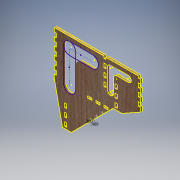
# Autodesk Inventor part: ArmSide
Saved by Autodesk Inventor 2019 (Build 230136000, 136)
## iProperties
Created: 2019-01-17
Part Number: ArmSide
Material: Wood (Birch)
Document SubType Name: Modeling
Designer: nxgam
Density: 0.55 g/cm^3
Appearance: Birch - Natural Polished
Mass: 65.7637 g
Surface Area: 562.081 cm^2
Volume: 119.57 cm^3
Author: nxgam
Autodesk Inventor part; units mm, degrees
(part 1 of 2)
ref_plane "YZ Plane" through (0, 0, 0) normal (1, 0, 0) x (0, 1, 0)
ref_plane "XZ Plane" through (0, 0, 0) normal (0, 1, 0) x (-1, 0, 0)
ref_plane "XY Plane" through (0, 0, 0) normal (0, 0, 1) x (1, 0, 0)
sketch "Sketch1" plane through (0, 0, 0) normal (0, 0, 1) x (1, 0, 0)
  line L0 (0, 0) -> (76.2, 0)
  line L1 (76.2, 0) -> (76.2, 579.12)
  line L2 (76.2, 579.12) -> (0, 579.12)
  line L3 (0, 579.12) -> (0, 0)
  line L4 (0, 568.96) -> (5.08, 568.96)
  line L5 (5.08, 568.96) -> (5.08, 558.8)
  line L6 (5.08, 558.8) -> (0, 558.8)
  line L7 (0, 558.8) -> (0, 568.96)
  line L8 (0, 548.64) -> (5.08, 548.64)
  line L9 (5.08, 548.64) -> (5.08, 538.48)
  line L10 (5.08, 538.48) -> (0, 538.48)
  line L11 (0, 538.48) -> (0, 548.64)
  line L12 (0, 558.8) -> (0, -20.32)
  line L13 (0, 528.32) -> (5.08, 528.32)
  line L14 (5.08, 528.32) -> (5.08, 518.16)
  line L15 (5.08, 518.16) -> (0, 518.16)
  line L16 (0, 518.16) -> (0, 528.32)
  line L17 (0, 538.48) -> (0, -40.64)
  line L18 (0, 508) -> (5.08, 508)
  line L19 (5.08, 508) -> (5.08, 497.84)
  line L20 (5.08, 497.84) -> (0, 497.84)
  line L21 (0, 497.84) -> (0, 508)
  line L22 (0, 518.16) -> (0, -60.96)
  line L23 (0, 487.68) -> (5.08, 487.68)
  line L24 (5.08, 487.68) -> (5.08, 477.52)
  line L25 (5.08, 477.52) -> (0, 477.52)
  line L26 (0, 477.52) -> (0, 487.68)
  line L27 (0, 497.84) -> (0, -81.28)
  line L28 (0, 467.36) -> (5.08, 467.36)
  line L29 (5.08, 467.36) -> (5.08, 457.2)
  line L30 (5.08, 457.2) -> (0, 457.2)
  line L31 (0, 457.2) -> (0, 467.36)
  line L32 (0, 477.52) -> (0, -101.6)
  line L33 (0, 447.04) -> (5.08, 447.04)
  line L34 (5.08, 447.04) -> (5.08, 436.88)
  line L35 (5.08, 436.88) -> (0, 436.88)
  line L36 (0, 436.88) -> (0, 447.04)
  line L37 (0, 457.2) -> (0, -121.92)
  line L38 (0, 426.72) -> (5.08, 426.72)
  line L39 (5.08, 426.72) -> (5.08, 416.56)
  line L40 (5.08, 416.56) -> (0, 416.56)
  line L41 (0, 416.56) -> (0, 426.72)
  line L42 (0, 436.88) -> (0, -142.24)
  line L43 (0, 406.4) -> (5.08, 406.4)
  line L44 (5.08, 406.4) -> (5.08, 396.24)
  line L45 (5.08, 396.24) -> (0, 396.24)
  line L46 (0, 396.24) -> (0, 406.4)
  line L47 (0, 416.56) -> (0, -162.56)
  line L48 (0, 386.08) -> (5.08, 386.08)
  line L49 (5.08, 386.08) -> (5.08, 375.92)
  line L50 (5.08, 375.92) -> (0, 375.92)
  line L51 (0, 375.92) -> (0, 386.08)
  line L52 (0, 396.24) -> (0, -182.88)
  line L53 (0, 365.76) -> (5.08, 365.76)
  line L54 (5.08, 365.76) -> (5.08, 355.6)
  line L55 (5.08, 355.6) -> (0, 355.6)
  line L56 (0, 355.6) -> (0, 365.76)
  line L57 (0, 375.92) -> (0, -203.2)
  line L58 (0, 345.44) -> (5.08, 345.44)
  line L59 (5.08, 345.44) -> (5.08, 335.28)
  line L60 (5.08, 335.28) -> (0, 335.28)
  line L61 (0, 335.28) -> (0, 345.44)
  line L62 (0, 355.6) -> (0, -223.52)
  line L63 (0, 325.12) -> (5.08, 325.12)
  line L64 (5.08, 325.12) -> (5.08, 314.96)
  line L65 (5.08, 314.96) -> (0, 314.96)
  line L66 (0, 314.96) -> (0, 325.12)
  line L67 (0, 335.28) -> (0, -243.84)
  line L68 (0, 304.8) -> (5.08, 304.8)
  line L69 (5.08, 304.8) -> (5.08, 294.64)
  line L70 (5.08, 294.64) -> (0, 294.64)
  line L71 (0, 294.64) -> (0, 304.8)
  line L72 (0, 314.96) -> (0, -264.16)
  line L73 (0, 284.48) -> (5.08, 284.48)
  line L74 (5.08, 284.48) -> (5.08, 274.32)
  line L75 (5.08, 274.32) -> (0, 274.32)
  line L76 (0, 274.32) -> (0, 284.48)
  line L77 (0, 294.64) -> (0, -284.48)
  line L78 (0, 264.16) -> (5.08, 264.16)
  line L79 (5.08, 264.16) -> (5.08, 254)
  line L80 (5.08, 254) -> (0, 254)
  line L81 (0, 254) -> (0, 264.16)
  line L82 (0, 274.32) -> (0, -304.8)
  line L83 (0, 243.84) -> (5.08, 243.84)
  line L84 (5.08, 243.84) -> (5.08, 233.68)
  line L85 (5.08, 233.68) -> (0, 233.68)
  line L86 (0, 233.68) -> (0, 243.84)
  line L87 (0, 254) -> (0, -325.12)
  line L88 (0, 223.52) -> (5.08, 223.52)
  line L89 (5.08, 223.52) -> (5.08, 213.36)
  line L90 (5.08, 213.36) -> (0, 213.36)
  line L91 (0, 213.36) -> (0, 223.52)
  line L92 (0, 233.68) -> (0, -345.44)
  line L93 (0, 203.2) -> (5.08, 203.2)
  line L94 (5.08, 203.2) -> (5.08, 193.04)
  line L95 (5.08, 193.04) -> (0, 193.04)
  line L96 (0, 193.04) -> (0, 203.2)
  line L97 (0, 213.36) -> (0, -365.76)
  line L98 (0, 182.88) -> (5.08, 182.88)
  line L99 (5.08, 182.88) -> (5.08, 172.72)
  line L100 (5.08, 172.72) -> (0, 172.72)
  line L101 (0, 172.72) -> (0, 182.88)
  line L102 (0, 193.04) -> (0, -386.08)
  line L103 (0, 162.56) -> (5.08, 162.56)
  line L104 (5.08, 162.56) -> (5.08, 152.4)
  line L105 (5.08, 152.4) -> (0, 152.4)
  line L106 (0, 152.4) -> (0, 162.56)
  line L107 (0, 172.72) -> (0, -406.4)
  line L108 (0, 142.24) -> (5.08, 142.24)
  line L109 (5.08, 142.24) -> (5.08, 132.08)
  line L110 (5.08, 132.08) -> (0, 132.08)
  line L111 (0, 132.08) -> (0, 142.24)
  line L112 (0, 152.4) -> (0, -426.72)
  line L113 (0, 121.92) -> (5.08, 121.92)
  line L114 (5.08, 121.92) -> (5.08, 111.76)
  line L115 (5.08, 111.76) -> (0, 111.76)
  line L116 (0, 111.76) -> (0, 121.92)
  line L117 (0, 132.08) -> (0, -447.04)
  line L118 (0, 101.6) -> (5.08, 101.6)
  line L119 (5.08, 101.6) -> (5.08, 91.44)
  line L120 (5.08, 91.44) -> (0, 91.44)
  line L121 (0, 91.44) -> (0, 101.6)
  line L122 (0, 111.76) -> (0, -467.36)
  line L123 (0, 81.28) -> (5.08, 81.28)
  line L124 (5.08, 81.28) -> (5.08, 71.12)
  line L125 (5.08, 71.12) -> (0, 71.12)
  line L126 (0, 71.12) -> (0, 81.28)
  line L127 (0, 91.44) -> (0, -487.68)
  line L128 (0, 60.96) -> (5.08, 60.96)
  line L129 (5.08, 60.96) -> (5.08, 50.8)
  line L130 (5.08, 50.8) -> (0, 50.8)
  line L131 (0, 50.8) -> (0, 60.96)
  line L132 (0, 71.12) -> (0, -508)
  line L133 (0, 40.64) -> (5.08, 40.64)
  line L134 (5.08, 40.64) -> (5.08, 30.48)
  line L135 (5.08, 30.48) -> (0, 30.48)
  line L136 (0, 30.48) -> (0, 40.64)
  line L137 (0, 50.8) -> (0, -528.32)
  line L138 (0, 20.32) -> (5.08, 20.32)
  line L139 (5.08, 20.32) -> (5.08, 10.16)
  line L140 (5.08, 10.16) -> (0, 10.16)
  line L141 (0, 10.16) -> (0, 20.32)
  line L142 (0, 30.48) -> (0, -548.64)
  line L143 (0, 0) -> (5.08, 0)
  line L144 (5.08, 0) -> (5.08, -10.16)
  line L145 (5.08, -10.16) -> (0, -10.16)
  line L146 (0, -10.16) -> (0, 0)
  line L147 (0, 10.16) -> (0, -568.96)
  line L148 (0, -20.32) -> (5.08, -20.32)
  line L149 (5.08, -20.32) -> (5.08, -30.48)
  line L150 (5.08, -30.48) -> (0, -30.48)
  line L151 (0, -30.48) -> (0, -20.32)
  line L152 (0, -10.16) -> (0, -589.28)
  line L153 (38.1, 579.12) -> (38.1, 0) construction
  line L154 (76.2, 579.12) -> (76.2, 0) construction
  line L155 (76.2, 568.96) -> (71.12, 568.96) construction
  line L156 (71.12, 568.96) -> (71.12, 558.8) construction
  line L157 (71.12, 558.8) -> (76.2, 558.8) construction
  line L158 (76.2, 558.8) -> (76.2, 568.96) construction
  line L159 (76.2, 548.64) -> (71.12, 548.64) construction
  line L160 (71.12, 548.64) -> (71.12, 538.48) construction
  line L161 (71.12, 538.48) -> (76.2, 538.48) construction
  line L162 (76.2, 538.48) -> (76.2, 548.64) construction
  line L163 (76.2, 558.8) -> (76.2, -20.32) construction
  line L164 (76.2, 528.32) -> (71.12, 528.32) construction
  line L165 (71.12, 528.32) -> (71.12, 518.16) construction
  line L166 (71.12, 518.16) -> (76.2, 518.16) construction
  line L167 (76.2, 518.16) -> (76.2, 528.32) construction
  line L168 (76.2, 538.48) -> (76.2, -40.64) construction
  line L169 (76.2, 508) -> (71.12, 508) construction
  line L170 (71.12, 508) -> (71.12, 497.84) construction
  line L171 (71.12, 497.84) -> (76.2, 497.84) construction
  line L172 (76.2, 497.84) -> (76.2, 508) construction
  line L173 (76.2, 518.16) -> (76.2, -60.96) construction
  line L174 (76.2, 487.68) -> (71.12, 487.68) construction
  line L175 (71.12, 487.68) -> (71.12, 477.52) construction
  line L176 (71.12, 477.52) -> (76.2, 477.52) construction
  line L177 (76.2, 477.52) -> (76.2, 487.68) construction
  line L178 (76.2, 497.84) -> (76.2, -81.28) construction
  line L179 (76.2, 467.36) -> (71.12, 467.36) construction
  line L180 (71.12, 467.36) -> (71.12, 457.2) construction
  line L181 (71.12, 457.2) -> (76.2, 457.2) construction
  line L182 (76.2, 457.2) -> (76.2, 467.36) construction
  line L183 (76.2, 477.52) -> (76.2, -101.6)
  line L184 (76.2, 447.04) -> (71.12, 447.04) construction
  line L185 (71.12, 447.04) -> (71.12, 436.88) construction
  line L186 (71.12, 436.88) -> (76.2, 436.88) construction
  line L187 (76.2, 436.88) -> (76.2, 447.04) construction
  line L188 (76.2, 457.2) -> (76.2, -121.92) construction
  line L189 (76.2, 426.72) -> (71.12, 426.72) construction
  line L190 (71.12, 426.72) -> (71.12, 416.56) construction
  line L191 (71.12, 416.56) -> (76.2, 416.56) construction
  line L192 (76.2, 416.56) -> (76.2, 426.72) construction
  line L193 (76.2, 436.88) -> (76.2, -142.24) construction
  line L194 (76.2, 406.4) -> (71.12, 406.4) construction
  line L195 (71.12, 406.4) -> (71.12, 396.24) construction
  line L196 (71.12, 396.24) -> (76.2, 396.24) construction
  line L197 (76.2, 396.24) -> (76.2, 406.4) construction
  line L198 (76.2, 416.56) -> (76.2, -162.56) construction
  line L199 (76.2, 386.08) -> (71.12, 386.08) construction
  line L200 (71.12, 386.08) -> (71.12, 375.92) construction
  line L201 (71.12, 375.92) -> (76.2, 375.92) construction
  line L202 (76.2, 375.92) -> (76.2, 386.08) construction
  line L203 (76.2, 396.24) -> (76.2, -182.88) construction
  line L204 (76.2, 365.76) -> (71.12, 365.76) construction
  line L205 (71.12, 365.76) -> (71.12, 355.6) construction
  line L206 (71.12, 355.6) -> (76.2, 355.6) construction
  line L207 (76.2, 355.6) -> (76.2, 365.76) construction
  line L208 (76.2, 375.92) -> (76.2, -203.2) construction
  line L209 (76.2, 345.44) -> (71.12, 345.44) construction
  line L210 (71.12, 345.44) -> (71.12, 335.28) construction
  line L211 (71.12, 335.28) -> (76.2, 335.28) construction
  line L212 (76.2, 335.28) -> (76.2, 345.44) construction
  line L213 (76.2, 325.12) -> (71.12, 325.12) construction
  line L214 (71.12, 325.12) -> (71.12, 314.96) construction
  line L215 (71.12, 314.96) -> (76.2, 314.96) construction
  line L216 (76.2, 314.96) -> (76.2, 325.12) construction
  line L217 (76.2, 304.8) -> (71.12, 304.8) construction
  line L218 (71.12, 304.8) -> (71.12, 294.64) construction
  line L219 (71.12, 294.64) -> (76.2, 294.64) construction
  line L220 (76.2, 294.64) -> (76.2, 304.8) construction
  line L221 (76.2, 284.48) -> (71.12, 284.48) construction
  line L222 (71.12, 284.48) -> (71.12, 274.32) construction
  line L223 (71.12, 274.32) -> (76.2, 274.32) construction
  line L224 (76.2, 274.32) -> (76.2, 284.48) construction
  line L225 (76.2, 264.16) -> (71.12, 264.16) construction
  line L226 (71.12, 264.16) -> (71.12, 254) construction
  line L227 (71.12, 254) -> (76.2, 254) construction
  line L228 (76.2, 254) -> (76.2, 264.16) construction
  line L229 (76.2, 243.84) -> (71.12, 243.84) construction
  line L230 (71.12, 243.84) -> (71.12, 233.68) construction
  line L231 (71.12, 233.68) -> (76.2, 233.68) construction
  line L232 (76.2, 233.68) -> (76.2, 243.84) construction
  line L233 (76.2, 223.52) -> (71.12, 223.52) construction
  line L234 (71.12, 223.52) -> (71.12, 213.36) construction
  line L235 (71.12, 213.36) -> (76.2, 213.36) construction
  line L236 (76.2, 213.36) -> (76.2, 223.52) construction
  line L237 (76.2, 203.2) -> (71.12, 203.2) construction
  line L238 (71.12, 203.2) -> (71.12, 193.04) construction
  line L239 (71.12, 193.04) -> (76.2, 193.04) construction
  line L240 (76.2, 193.04) -> (76.2, 203.2) construction
  line L241 (76.2, 182.88) -> (71.12, 182.88) construction
  line L242 (71.12, 182.88) -> (71.12, 172.72) construction
  line L243 (71.12, 172.72) -> (76.2, 172.72) construction
  line L244 (76.2, 172.72) -> (76.2, 182.88) construction
  line L245 (76.2, 162.56) -> (71.12, 162.56) construction
  line L246 (71.12, 162.56) -> (71.12, 152.4) construction
  line L247 (71.12, 152.4) -> (76.2, 152.4) construction
  line L248 (76.2, 152.4) -> (76.2, 162.56) construction
  line L249 (76.2, 142.24) -> (71.12, 142.24) construction
  line L250 (71.12, 142.24) -> (71.12, 132.08) construction
  line L251 (71.12, 132.08) -> (76.2, 132.08) construction
  line L252 (76.2, 132.08) -> (76.2, 142.24) construction
  line L253 (76.2, 121.92) -> (71.12, 121.92) construction
  line L254 (71.12, 121.92) -> (71.12, 111.76) construction
  line L255 (71.12, 111.76) -> (76.2, 111.76) construction
  line L256 (76.2, 111.76) -> (76.2, 121.92) construction
  line L257 (76.2, 101.6) -> (71.12, 101.6) construction
  line L258 (71.12, 101.6) -> (71.12, 91.44) construction
  line L259 (71.12, 91.44) -> (76.2, 91.44) construction
  line L260 (76.2, 91.44) -> (76.2, 101.6) construction
  line L261 (76.2, 81.28) -> (71.12, 81.28) construction
  line L262 (71.12, 81.28) -> (71.12, 71.12) construction
  line L263 (71.12, 71.12) -> (76.2, 71.12) construction
  line L264 (76.2, 71.12) -> (76.2, 81.28) construction
  line L265 (76.2, 60.96) -> (71.12, 60.96) construction
  line L266 (71.12, 60.96) -> (71.12, 50.8) construction
  line L267 (71.12, 50.8) -> (76.2, 50.8) construction
  line L268 (76.2, 50.8) -> (76.2, 60.96) construction
  line L269 (76.2, 40.64) -> (71.12, 40.64) construction
  line L270 (71.12, 40.64) -> (71.12, 30.48) construction
  line L271 (71.12, 30.48) -> (76.2, 30.48) construction
  line L272 (76.2, 30.48) -> (76.2, 40.64) construction
  line L273 (76.2, 20.32) -> (71.12, 20.32) construction
  line L274 (71.12, 20.32) -> (71.12, 10.16) construction
  line L275 (71.12, 10.16) -> (76.2, 10.16) construction
  line L276 (76.2, 10.16) -> (76.2, 20.32) construction
  line L277 (76.2, 0) -> (71.12, 0) construction
  line L278 (71.12, 0) -> (71.12, -10.16) construction
  line L279 (71.12, -10.16) -> (76.2, -10.16) construction
  line L280 (76.2, -10.16) -> (76.2, 0) construction
  line L281 (76.2, -20.32) -> (71.12, -20.32) construction
  line L282 (71.12, -20.32) -> (71.12, -30.48) construction
  line L283 (71.12, -30.48) -> (76.2, -30.48) construction
  line L284 (76.2, -30.48) -> (76.2, -20.32) construction
  dimension "d0" = 76.2
  dimension "d1" = 579.12
  dimension "d2" = 5.08
  dimension "d3" = 10.16
  dimension "d4" = 10.16
  dimension "d7" = 20.32
  constraints: 570 end point, 160 symmetric about line, 41 point on line, 4 parallel, 2 horizontal, 2 midpoint, 2 perpendicular, 1 collinear, 1 vertical, 318 other
  measures "d0" distance of L2.end L1.end
  measures "d1" distance of L1.end L0.end
  measures "d2" distance of L5.end L6.end
  measures "d3" distance of L4.end L5.end
  measures "d4" distance between parallel lines of L2 L4
  measures "d7" distance of L4.start L8.start
extrude "Extrusion2" add sketch "Sketch1" along normal blind 5.08 contours L3 L140 L139 L138 L135 L134 L133 L130 L129 L128 L125 L124 L123 L120 L119 L118 L115 L114 L113 L110 L109 L108 L105 L104 L103 L100 L99 L98 L95 L94 L93 L90 L89 L88 L85 L84 L83 L80 L79 L78 L75 L74 L73 L70 L69 L68 L65 L64 L63 L60 L59 L58 L55 L54 L53 L50 L49 L48 L45 L44 L43 L40 L39 L38 L35 L34 L33 L30 L29 L28 L25 L24 L23 L20 L19 L18 L15 L14 L13 L10 L9 L8 L6 L5 L4 L2 L1 L0
sketch "Sketch2" plane through (0, 0, 5.08) normal (0, 0, 1) x (1, 0, 0)
  line L0 (0, 20.32) -> (5.08, 20.32) projected
  line L1 (5.08, 20.32) -> (5.08, 10.16) projected
  line L2 (5.08, 10.16) -> (0, 10.16) projected
  line L3 (0, 10.16) -> (0, 0) projected
  line L4 (0, 0) -> (76.2, 0) projected
  line L5 (76.2, 0) -> (76.2, 579.12) projected
  line L6 (76.2, 579.12) -> (0, 579.12) projected
  line L7 (0, 579.12) -> (0, 568.96) projected
  line L8 (0, 568.96) -> (5.08, 568.96) projected
  line L9 (5.08, 568.96) -> (5.08, 558.8) projected
  line L10 (5.08, 558.8) -> (0, 558.8) projected
  line L11 (0, 558.8) -> (0, 548.64) projected
  line L12 (0, 548.64) -> (5.08, 548.64) projected
  line L13 (5.08, 548.64) -> (5.08, 538.48) projected
  line L14 (5.08, 538.48) -> (0, 538.48) projected
  line L15 (0, 538.48) -> (0, 528.32) projected
  line L16 (0, 528.32) -> (5.08, 528.32) projected
  line L17 (5.08, 528.32) -> (5.08, 518.16) projected
  line L18 (5.08, 518.16) -> (0, 518.16) projected
  line L19 (0, 518.16) -> (0, 508) projected
  line L20 (0, 508) -> (5.08, 508) projected
  line L21 (5.08, 508) -> (5.08, 497.84) projected
  line L22 (5.08, 497.84) -> (0, 497.84) projected
  line L23 (0, 497.84) -> (0, 487.68) projected
  line L24 (0, 487.68) -> (5.08, 487.68) projected
  line L25 (5.08, 487.68) -> (5.08, 477.52) projected
  line L26 (5.08, 477.52) -> (0, 477.52) projected
  line L27 (0, 477.52) -> (0, 467.36) projected
  line L28 (0, 467.36) -> (5.08, 467.36) projected
  line L29 (5.08, 467.36) -> (5.08, 457.2) projected
  line L30 (5.08, 457.2) -> (0, 457.2) projected
  line L31 (0, 457.2) -> (0, 447.04) projected
  line L32 (0, 447.04) -> (5.08, 447.04) projected
  line L33 (5.08, 447.04) -> (5.08, 436.88) projected
  line L34 (5.08, 436.88) -> (0, 436.88) projected
  line L35 (0, 436.88) -> (0, 426.72) projected
  line L36 (0, 426.72) -> (5.08, 426.72) projected
  line L37 (5.08, 426.72) -> (5.08, 416.56) projected
  line L38 (5.08, 416.56) -> (0, 416.56) projected
  line L39 (0, 416.56) -> (0, 406.4) projected
  line L40 (0, 406.4) -> (5.08, 406.4) projected
  line L41 (5.08, 406.4) -> (5.08, 396.24) projected
  line L42 (5.08, 396.24) -> (0, 396.24) projected
  line L43 (0, 396.24) -> (0, 386.08) projected
  line L44 (0, 386.08) -> (5.08, 386.08) projected
  line L45 (5.08, 386.08) -> (5.08, 375.92) projected
  line L46 (5.08, 375.92) -> (0, 375.92) projected
  line L47 (0, 375.92) -> (0, 365.76) projected
  line L48 (0, 365.76) -> (5.08, 365.76) projected
  line L49 (5.08, 365.76) -> (5.08, 355.6) projected
  line L50 (5.08, 355.6) -> (0, 355.6) projected
  line L51 (0, 355.6) -> (0, 345.44) projected
  line L52 (0, 345.44) -> (5.08, 345.44) projected
  line L53 (5.08, 345.44) -> (5.08, 335.28) projected
  line L54 (5.08, 335.28) -> (0, 335.28) projected
  line L55 (0, 335.28) -> (0, 325.12) projected
  line L56 (0, 325.12) -> (5.08, 325.12) projected
  line L57 (5.08, 325.12) -> (5.08, 314.96) projected
  line L58 (5.08, 314.96) -> (0, 314.96) projected
  line L59 (0, 314.96) -> (0, 304.8) projected
  line L60 (0, 304.8) -> (5.08, 304.8) projected
  line L61 (5.08, 304.8) -> (5.08, 294.64) projected
  line L62 (5.08, 294.64) -> (0, 294.64) projected
  line L63 (0, 294.64) -> (0, 284.48) projected
  line L64 (0, 284.48) -> (5.08, 284.48) projected
  line L65 (5.08, 284.48) -> (5.08, 274.32) projected
  line L66 (5.08, 274.32) -> (0, 274.32) projected
  line L67 (0, 274.32) -> (0, 264.16) projected
  line L68 (0, 264.16) -> (5.08, 264.16) projected
  line L69 (5.08, 264.16) -> (5.08, 254) projected
  line L70 (5.08, 254) -> (0, 254) projected
  line L71 (0, 254) -> (0, 243.84) projected
  line L72 (0, 243.84) -> (5.08, 243.84) projected
  line L73 (5.08, 243.84) -> (5.08, 233.68) projected
  line L74 (5.08, 233.68) -> (0, 233.68) projected
  line L75 (0, 233.68) -> (0, 223.52) projected
  line L76 (0, 223.52) -> (5.08, 223.52) projected
  line L77 (5.08, 223.52) -> (5.08, 213.36) projected
  line L78 (5.08, 213.36) -> (0, 213.36) projected
  line L79 (0, 213.36) -> (0, 203.2) projected
  line L80 (0, 203.2) -> (5.08, 203.2) projected
  line L81 (5.08, 203.2) -> (5.08, 193.04) projected
  line L82 (5.08, 193.04) -> (0, 193.04) projected
  line L83 (0, 193.04) -> (0, 182.88) projected
  line L84 (0, 182.88) -> (5.08, 182.88) projected
  line L85 (5.08, 182.88) -> (5.08, 172.72) projected
  line L86 (5.08, 172.72) -> (0, 172.72) projected
  line L87 (0, 172.72) -> (0, 162.56) projected
  line L88 (0, 162.56) -> (5.08, 162.56) projected
  line L89 (5.08, 162.56) -> (5.08, 152.4) projected
  line L90 (5.08, 152.4) -> (0, 152.4) projected
  line L91 (0, 152.4) -> (0, 142.24) projected
  line L92 (0, 142.24) -> (5.08, 142.24) projected
  line L93 (5.08, 142.24) -> (5.08, 132.08) projected
  line L94 (5.08, 132.08) -> (0, 132.08) projected
  line L95 (0, 132.08) -> (0, 121.92) projected
  line L96 (0, 121.92) -> (5.08, 121.92) projected
  line L97 (5.08, 121.92) -> (5.08, 111.76) projected
  line L98 (5.08, 111.76) -> (0, 111.76) projected
  line L99 (0, 111.76) -> (0, 101.6) projected
  line L100 (0, 101.6) -> (5.08, 101.6) projected
  line L101 (5.08, 101.6) -> (5.08, 91.44) projected
  line L102 (5.08, 91.44) -> (0, 91.44) projected
  line L103 (0, 91.44) -> (0, 81.28) projected
  line L104 (0, 81.28) -> (5.08, 81.28) projected
  line L105 (5.08, 81.28) -> (5.08, 71.12) projected
  line L106 (5.08, 71.12) -> (0, 71.12) projected
  line L107 (0, 71.12) -> (0, 60.96) projected
  line L108 (0, 60.96) -> (5.08, 60.96) projected
  line L109 (5.08, 60.96) -> (5.08, 50.8) projected
  line L110 (5.08, 50.8) -> (0, 50.8) projected
  line L111 (0, 50.8) -> (0, 40.64) projected
  line L112 (0, 40.64) -> (5.08, 40.64) projected
  line L113 (5.08, 40.64) -> (5.08, 30.48) projected
  line L114 (5.08, 30.48) -> (0, 30.48) projected
  line L115 (0, 30.48) -> (0, 20.32) projected
  line L116 (76.2, 579.12) -> (215.9, 187.96)
  line L117 (215.9, 187.96) -> (215.9, 35.56)
  line L118 (0, 0) -> (76.2, 0) projected
  line L119 (215.9, 35.56) -> (76.2, 0)
  dimension "d18" = 152.4
  dimension "d19" = 35.56
  dimension "d20" = 139.7
  constraints: 6 end point, 1 vertical
  measures "d18" distance of L116.end L117.end
  measures "d19" distance from line of L117.end L118
  measures "d20" distance between parallel lines of L117 L5
extrude "Extrusion3" add sketch "Sketch2" against normal blind 5.08 contours L5 L116 L117 L119
sketch "Sketch3" plane through (0, 0, 5.08) normal (0, 0, 1) x (1, 0, 0)
  line L0 (0, 20.32) -> (5.08, 20.32) projected
  line L1 (5.08, 20.32) -> (5.08, 10.16) projected
  line L2 (5.08, 10.16) -> (0, 10.16) projected
  line L3 (0, 10.16) -> (0, 0) projected
  line L4 (0, 0) -> (76.2, 0) projected
  line L5 (76.2, 0) -> (215.9, 35.56) projected
  line L6 (215.9, 35.56) -> (215.9, 187.96) projected
  line L7 (215.9, 187.96) -> (76.2, 579.12) projected
  line L8 (76.2, 579.12) -> (0, 579.12) projected
  line L9 (0, 579.12) -> (0, 568.96) projected
  line L10 (0, 568.96) -> (5.08, 568.96) projected
  line L11 (5.08, 568.96) -> (5.08, 558.8) projected
  line L12 (5.08, 558.8) -> (0, 558.8) projected
  line L13 (0, 558.8) -> (0, 548.64) projected
  line L14 (0, 548.64) -> (5.08, 548.64) projected
  line L15 (5.08, 548.64) -> (5.08, 538.48) projected
  line L16 (5.08, 538.48) -> (0, 538.48) projected
  line L17 (0, 538.48) -> (0, 528.32) projected
  line L18 (0, 528.32) -> (5.08, 528.32) projected
  line L19 (5.08, 528.32) -> (5.08, 518.16) projected
  line L20 (5.08, 518.16) -> (0, 518.16) projected
  line L21 (0, 518.16) -> (0, 508) projected
  line L22 (0, 508) -> (5.08, 508) projected
  line L23 (5.08, 508) -> (5.08, 497.84) projected
  line L24 (5.08, 497.84) -> (0, 497.84) projected
  line L25 (0, 497.84) -> (0, 487.68) projected
  line L26 (0, 487.68) -> (5.08, 487.68) projected
  line L27 (5.08, 487.68) -> (5.08, 477.52) projected
  line L28 (5.08, 477.52) -> (0, 477.52) projected
  line L29 (0, 477.52) -> (0, 467.36) projected
  line L30 (0, 467.36) -> (5.08, 467.36) projected
  line L31 (5.08, 467.36) -> (5.08, 457.2) projected
  line L32 (5.08, 457.2) -> (0, 457.2) projected
  line L33 (0, 457.2) -> (0, 447.04) projected
  line L34 (0, 447.04) -> (5.08, 447.04) projected
  line L35 (5.08, 447.04) -> (5.08, 436.88) projected
  line L36 (5.08, 436.88) -> (0, 436.88) projected
  line L37 (0, 436.88) -> (0, 426.72) projected
  line L38 (0, 426.72) -> (5.08, 426.72) projected
  line L39 (5.08, 426.72) -> (5.08, 416.56) projected
  line L40 (5.08, 416.56) -> (0, 416.56) projected
  line L41 (0, 416.56) -> (0, 406.4) projected
  line L42 (0, 406.4) -> (5.08, 406.4) projected
  line L43 (5.08, 406.4) -> (5.08, 396.24) projected
  line L44 (5.08, 396.24) -> (0, 396.24) projected
  line L45 (0, 396.24) -> (0, 386.08) projected
  line L46 (0, 386.08) -> (5.08, 386.08) projected
  line L47 (5.08, 386.08) -> (5.08, 375.92) projected
  line L48 (5.08, 375.92) -> (0, 375.92) projected
  line L49 (0, 375.92) -> (0, 365.76) projected
  line L50 (0, 365.76) -> (5.08, 365.76) projected
  line L51 (5.08, 365.76) -> (5.08, 355.6) projected
  line L52 (5.08, 355.6) -> (0, 355.6) projected
  line L53 (0, 355.6) -> (0, 345.44) projected
  line L54 (0, 345.44) -> (5.08, 345.44) projected
  line L55 (5.08, 345.44) -> (5.08, 335.28) projected
  line L56 (5.08, 335.28) -> (0, 335.28) projected
  line L57 (0, 335.28) -> (0, 325.12) projected
  line L58 (0, 325.12) -> (5.08, 325.12) projected
  line L59 (5.08, 325.12) -> (5.08, 314.96) projected
  line L60 (5.08, 314.96) -> (0, 314.96) projected
  line L61 (0, 314.96) -> (0, 304.8) projected
  line L62 (0, 304.8) -> (5.08, 304.8) projected
  line L63 (5.08, 304.8) -> (5.08, 294.64) projected
  line L64 (5.08, 294.64) -> (0, 294.64) projected
  line L65 (0, 294.64) -> (0, 284.48) projected
  line L66 (0, 284.48) -> (5.08, 284.48) projected
  line L67 (5.08, 284.48) -> (5.08, 274.32) projected
  line L68 (5.08, 274.32) -> (0, 274.32) projected
  line L69 (0, 274.32) -> (0, 264.16) projected
  line L70 (0, 264.16) -> (5.08, 264.16) projected
  line L71 (5.08, 264.16) -> (5.08, 254) projected
  line L72 (5.08, 254) -> (0, 254) projected
  line L73 (0, 254) -> (0, 243.84) projected
  line L74 (0, 243.84) -> (5.08, 243.84) projected
  line L75 (5.08, 243.84) -> (5.08, 233.68) projected
  line L76 (5.08, 233.68) -> (0, 233.68) projected
  line L77 (0, 233.68) -> (0, 223.52) projected
  line L78 (0, 223.52) -> (5.08, 223.52) projected
  line L79 (5.08, 223.52) -> (5.08, 213.36) projected
  line L80 (5.08, 213.36) -> (0, 213.36) projected
  line L81 (0, 213.36) -> (0, 203.2) projected
  line L82 (0, 203.2) -> (5.08, 203.2) projected
  line L83 (5.08, 203.2) -> (5.08, 193.04) projected
  line L84 (5.08, 193.04) -> (0, 193.04) projected
  line L85 (0, 193.04) -> (0, 182.88) projected
  line L86 (0, 182.88) -> (5.08, 182.88) projected
  line L87 (5.08, 182.88) -> (5.08, 172.72) projected
  line L88 (5.08, 172.72) -> (0, 172.72) projected
  line L89 (0, 172.72) -> (0, 162.56) projected
  line L90 (0, 162.56) -> (5.08, 162.56) projected
  line L91 (5.08, 162.56) -> (5.08, 152.4) projected
  line L92 (5.08, 152.4) -> (0, 152.4) projected
  line L93 (0, 152.4) -> (0, 142.24) projected
  line L94 (0, 142.24) -> (5.08, 142.24) projected
  line L95 (5.08, 142.24) -> (5.08, 132.08) projected
  line L96 (5.08, 132.08) -> (0, 132.08) projected
  line L97 (0, 132.08) -> (0, 121.92) projected
  line L98 (0, 121.92) -> (5.08, 121.92) projected
  line L99 (5.08, 121.92) -> (5.08, 111.76) projected
  line L100 (5.08, 111.76) -> (0, 111.76) projected
  line L101 (0, 111.76) -> (0, 101.6) projected
  line L102 (0, 101.6) -> (5.08, 101.6) projected
  line L103 (5.08, 101.6) -> (5.08, 91.44) projected
  line L104 (5.08, 91.44) -> (0, 91.44) projected
  line L105 (0, 91.44) -> (0, 81.28) projected
  line L106 (0, 81.28) -> (5.08, 81.28) projected
  line L107 (5.08, 81.28) -> (5.08, 71.12) projected
  line L108 (5.08, 71.12) -> (0, 71.12) projected
  line L109 (0, 71.12) -> (0, 60.96) projected
  line L110 (0, 60.96) -> (5.08, 60.96) projected
  line L111 (5.08, 60.96) -> (5.08, 50.8) projected
  line L112 (5.08, 50.8) -> (0, 50.8) projected
  line L113 (0, 50.8) -> (0, 40.64) projected
  line L114 (0, 40.64) -> (5.08, 40.64) projected
  line L115 (5.08, 40.64) -> (5.08, 30.48) projected
  line L116 (5.08, 30.48) -> (0, 30.48) projected
  line L117 (0, 30.48) -> (0, 20.32) projected
  line L118 (0, 0) -> (20.32, -95.25)
  line L119 (20.32, -95.25) -> (42.545, -95.25)
  line L120 (42.545, -95.25) -> (147.32, 9.525)
  line L121 (147.32, 9.525) -> (169.545, 9.525)
  line L122 (169.545, 9.525) -> (215.9, 35.56)
  line L123 (210.82, 105.51) -> (210.82, 118.01) projected
  line L124 (133.48, 32.775) -> (133.48, 28.275) projected
  line L125 (157.48, 14.605) -> (152.4, 14.605) projected
  line L126 (152.4, 9.525) -> (152.4, 14.605) projected
  line L127 (157.48, 9.525) -> (152.4, 9.525) projected
  line L128 (157.48, 9.525) -> (157.48, 14.605) projected
  line L129 (157.48, 9.525) -> (157.48, 14.605)
  point P0 (210.82, 111.76)
  point P1 (133.48, 30.525)
  dimension "d22" = 22.225
  dimension "d23" = 95.25
  dimension "d24" = 20.32
  dimension "d45" = 81.235
  dimension "d46" = 9.525
  dimension "d47" = 68.58
  dimension "d98" = 135
  dimension "d99" = 22.225
  constraints: 12 end point, 2 midpoint, 1 horizontal, 1 parallel, 1 perpendicular
  measures "d22" distance of L120.end L121.end
  measures "d23" distance between parallel lines of L4 L119
  measures "d24" distance from line of L118.end L3
  measures "d45" vertical distance of point (210.82, 111.76) point (133.48, 30.525)
  measures "d46" distance between parallel lines of L4 L121
  measures "d47" distance from line of L6 L120.end
  measures "d98" angle of L120 L119
  measures "d99" distance of L118.end L119.end
extrude "Extrusion4" add sketch "Sketch3" against normal blind 5.08 contours L4 L5 L122 L121 L128 L125 L126 L120 L119 L118 | L121 L126 L125 L128
sketch "Sketch4" plane through (0, 0, 5.08) normal (0, 0, 1) x (1, 0, 0)
  line L0 (0, 20.32) -> (5.08, 20.32) projected
  line L1 (5.08, 20.32) -> (5.08, 10.16) projected
  line L2 (5.08, 10.16) -> (0, 10.16) projected
  line L3 (0, 10.16) -> (0, 0) projected
  line L4 (0, 0) -> (20.32, -95.25) projected
  line L5 (20.32, -95.25) -> (42.545, -95.25) projected
  line L6 (42.545, -95.25) -> (147.32, 9.525) projected
  line L7 (147.32, 9.525) -> (169.545, 9.525) projected
  line L8 (169.545, 9.525) -> (215.9, 35.56) projected
  line L9 (215.9, 35.56) -> (215.9, 187.96) projected
  line L10 (215.9, 187.96) -> (76.2, 579.12) projected
  line L11 (76.2, 579.12) -> (0, 579.12) projected
  line L12 (0, 579.12) -> (0, 568.96) projected
  line L13 (0, 568.96) -> (5.08, 568.96) projected
  line L14 (5.08, 568.96) -> (5.08, 558.8) projected
  line L15 (5.08, 558.8) -> (0, 558.8) projected
  line L16 (0, 558.8) -> (0, 548.64) projected
  line L17 (0, 548.64) -> (5.08, 548.64) projected
  line L18 (5.08, 548.64) -> (5.08, 538.48) projected
  line L19 (5.08, 538.48) -> (0, 538.48) projected
  line L20 (0, 538.48) -> (0, 528.32) projected
  line L21 (0, 528.32) -> (5.08, 528.32) projected
  line L22 (5.08, 528.32) -> (5.08, 518.16) projected
  line L23 (5.08, 518.16) -> (0, 518.16) projected
  line L24 (0, 518.16) -> (0, 508) projected
  line L25 (0, 508) -> (5.08, 508) projected
  line L26 (5.08, 508) -> (5.08, 497.84) projected
  line L27 (5.08, 497.84) -> (0, 497.84) projected
  line L28 (0, 497.84) -> (0, 487.68) projected
  line L29 (0, 487.68) -> (5.08, 487.68) projected
  line L30 (5.08, 487.68) -> (5.08, 477.52) projected
  line L31 (5.08, 477.52) -> (0, 477.52) projected
  line L32 (0, 477.52) -> (0, 467.36) projected
  line L33 (0, 467.36) -> (5.08, 467.36) projected
  line L34 (5.08, 467.36) -> (5.08, 457.2) projected
  line L35 (5.08, 457.2) -> (0, 457.2) projected
  line L36 (0, 457.2) -> (0, 447.04) projected
  line L37 (0, 447.04) -> (5.08, 447.04) projected
  line L38 (5.08, 447.04) -> (5.08, 436.88) projected
  line L39 (5.08, 436.88) -> (0, 436.88) projected
  line L40 (0, 436.88) -> (0, 426.72) projected
  line L41 (0, 426.72) -> (5.08, 426.72) projected
  line L42 (5.08, 426.72) -> (5.08, 416.56) projected
  line L43 (5.08, 416.56) -> (0, 416.56) projected
  line L44 (0, 416.56) -> (0, 406.4) projected
  line L45 (0, 406.4) -> (5.08, 406.4) projected
  line L46 (5.08, 406.4) -> (5.08, 396.24) projected
  line L47 (5.08, 396.24) -> (0, 396.24) projected
  line L48 (0, 396.24) -> (0, 386.08) projected
  line L49 (0, 386.08) -> (5.08, 386.08) projected
  line L50 (5.08, 386.08) -> (5.08, 375.92) projected
  line L51 (5.08, 375.92) -> (0, 375.92) projected
  line L52 (0, 375.92) -> (0, 365.76) projected
  line L53 (0, 365.76) -> (5.08, 365.76) projected
  line L54 (5.08, 365.76) -> (5.08, 355.6) projected
  line L55 (5.08, 355.6) -> (0, 355.6) projected
  line L56 (0, 355.6) -> (0, 345.44) projected
  line L57 (0, 345.44) -> (5.08, 345.44) projected
  line L58 (5.08, 345.44) -> (5.08, 335.28) projected
  line L59 (5.08, 335.28) -> (0, 335.28) projected
  line L60 (0, 335.28) -> (0, 325.12) projected
  line L61 (0, 325.12) -> (5.08, 325.12) projected
  line L62 (5.08, 325.12) -> (5.08, 314.96) projected
  line L63 (5.08, 314.96) -> (0, 314.96) projected
  line L64 (0, 314.96) -> (0, 304.8) projected
  line L65 (0, 304.8) -> (5.08, 304.8) projected
  line L66 (5.08, 304.8) -> (5.08, 294.64) projected
  line L67 (5.08, 294.64) -> (0, 294.64) projected
  line L68 (0, 294.64) -> (0, 284.48) projected
  line L69 (0, 284.48) -> (5.08, 284.48) projected
  line L70 (5.08, 284.48) -> (5.08, 274.32) projected
  line L71 (5.08, 274.32) -> (0, 274.32) projected
  line L72 (0, 274.32) -> (0, 264.16) projected
  line L73 (0, 264.16) -> (5.08, 264.16) projected
  line L74 (5.08, 264.16) -> (5.08, 254) projected
  line L75 (5.08, 254) -> (0, 254) projected
  line L76 (0, 254) -> (0, 243.84) projected
  line L77 (0, 243.84) -> (5.08, 243.84) projected
  line L78 (5.08, 243.84) -> (5.08, 233.68) projected
  line L79 (5.08, 233.68) -> (0, 233.68) projected
  line L80 (0, 233.68) -> (0, 223.52) projected
  line L81 (0, 223.52) -> (5.08, 223.52) projected
  line L82 (5.08, 223.52) -> (5.08, 213.36) projected
  line L83 (5.08, 213.36) -> (0, 213.36) projected
  line L84 (0, 213.36) -> (0, 203.2) projected
  line L85 (0, 203.2) -> (5.08, 203.2) projected
  line L86 (5.08, 203.2) -> (5.08, 193.04) projected
  line L87 (5.08, 193.04) -> (0, 193.04) projected
  line L88 (0, 193.04) -> (0, 182.88) projected
  line L89 (0, 182.88) -> (5.08, 182.88) projected
  line L90 (5.08, 182.88) -> (5.08, 172.72) projected
  line L91 (5.08, 172.72) -> (0, 172.72) projected
  line L92 (0, 172.72) -> (0, 162.56) projected
  line L93 (0, 162.56) -> (5.08, 162.56) projected
  line L94 (5.08, 162.56) -> (5.08, 152.4) projected
  line L95 (5.08, 152.4) -> (0, 152.4) projected
  line L96 (0, 152.4) -> (0, 142.24) projected
  line L97 (0, 142.24) -> (5.08, 142.24) projected
  line L98 (5.08, 142.24) -> (5.08, 132.08) projected
  line L99 (5.08, 132.08) -> (0, 132.08) projected
  line L100 (0, 132.08) -> (0, 121.92) projected
  line L101 (0, 121.92) -> (5.08, 121.92) projected
  line L102 (5.08, 121.92) -> (5.08, 111.76) projected
  line L103 (5.08, 111.76) -> (0, 111.76) projected
  line L104 (0, 111.76) -> (0, 101.6) projected
  line L105 (0, 101.6) -> (5.08, 101.6) projected
  line L106 (5.08, 101.6) -> (5.08, 91.44) projected
  line L107 (5.08, 91.44) -> (0, 91.44) projected
  line L108 (0, 91.44) -> (0, 81.28) projected
  line L109 (0, 81.28) -> (5.08, 81.28) projected
  line L110 (5.08, 81.28) -> (5.08, 71.12) projected
  line L111 (5.08, 71.12) -> (0, 71.12) projected
  line L112 (0, 71.12) -> (0, 60.96) projected
  line L113 (0, 60.96) -> (5.08, 60.96) projected
  line L114 (5.08, 60.96) -> (5.08, 50.8) projected
  line L115 (5.08, 50.8) -> (0, 50.8) projected
  line L116 (0, 50.8) -> (0, 40.64) projected
  line L117 (0, 40.64) -> (5.08, 40.64) projected
  line L118 (5.08, 40.64) -> (5.08, 30.48) projected
  line L119 (5.08, 30.48) -> (0, 30.48) projected
  line L120 (0, 30.48) -> (0, 20.32) projected
  line L121 (25.4, -90.17) -> (30.48, -90.17)
  line L122 (30.48, -90.17) -> (30.48, -80.01)
  line L123 (30.48, -80.01) -> (25.4, -80.01)
  line L124 (25.4, -80.01) -> (25.4, -90.17)
  line L125 (157.48, 14.605) -> (152.4, 14.605)
  line L126 (152.4, 14.605) -> (152.4, 24.765)
  line L127 (152.4, 24.765) -> (157.48, 24.765)
  line L128 (157.48, 24.765) -> (157.48, 14.605)
  line L129 (30.48, -59.69) -> (25.4, -59.69)
  line L130 (30.48, -69.85) -> (30.48, -59.69)
  line L131 (25.4, -59.69) -> (25.4, -69.85)
  line L132 (25.4, -69.85) -> (30.48, -69.85)
  line L133 (152.4, 34.925) -> (152.4, 45.085)
  line L134 (152.4, 45.085) -> (157.48, 45.085)
  line L135 (157.48, 34.925) -> (152.4, 34.925)
  line L136 (157.48, 45.085) -> (157.48, 34.925)
  line L137 (30.48, -39.37) -> (25.4, -39.37)
  line L138 (30.48, -49.53) -> (30.48, -39.37)
  line L139 (25.4, -39.37) -> (25.4, -49.53)
  line L140 (25.4, -49.53) -> (30.48, -49.53)
  line L141 (152.4, 55.245) -> (152.4, 65.405)
  line L142 (152.4, 65.405) -> (157.48, 65.405)
  line L143 (157.48, 55.245) -> (152.4, 55.245)
  line L144 (157.48, 65.405) -> (157.48, 55.245)
  line L145 (155.48, 28.275) -> (155.48, 32.775) projected
  line L146 (215.9, 118.01) -> (215.9, 105.51) projected
  line L147 (215.9, 118.01) -> (215.9, 105.51) projected
  line L148 (210.82, 105.51) -> (210.82, 118.01) projected
  point P0 (155.48, 30.525)
  point P1 (210.82, 111.76)
  dimension "d27" = 10.16
  dimension "d28" = 5.08
  dimension "d29" = 10.16
  dimension "d30" = 5.08
  dimension "d31" = 5.08
  dimension "d32" = 5.08
  dimension "d33" = 5.08
  dimension "d34" = 5.08
  dimension "d37" = 20.32
  dimension "d44" = 81.235
  constraints: 48 end point, 4 parallel, 2 horizontal, 2 midpoint, 2 perpendicular, 1 collinear, 1 vertical, 31 other
  measures "d27" distance of L125.end L126.end
  measures "d28" distance of L122.end L123.end
  measures "d29" distance of L121.end L122.end
  measures "d30" distance from line of L4.end L124
  measures "d31" distance between parallel lines of L5 L121
  measures "d32" distance of L126.end L127.end
  measures "d33" distance from line of L6.end L126
  measures "d34" distance between parallel lines of L7 L125
  measures "d37" distance of L122.end L129.start
  measures "d44" vertical distance of point (155.48, 30.525) point (210.82, 111.76)
extrude "Extrusion5" cut sketch "Sketch4" against normal blind 5.08 contours L124 L123 L122 L121 | L125 L126 L127 L128 | L130 L132 L131 L129 | L133 L134 L136 L135 | L138 L140 L139 L137 | L141 L142 L144 L143
sketch "Sketch5" plane through (0, 0, 5.08) normal (0, 0, 1) x (1, 0, 0)
  line L0 (215.9, 167.64) -> (210.82, 167.64)
  line L1 (210.82, 167.64) -> (210.82, 177.8)
  line L2 (210.82, 177.8) -> (215.9, 177.8)
  line L3 (215.9, 177.8) -> (215.9, 167.64)
  line L4 (215.9, 147.32) -> (210.82, 147.32)
  line L5 (210.82, 147.32) -> (210.82, 157.48)
  line L6 (210.82, 157.48) -> (215.9, 157.48)
  line L7 (215.9, 157.48) -> (215.9, 147.32)
  line L8 (215.9, 127) -> (210.82, 127)
  line L9 (210.82, 127) -> (210.82, 137.16)
  line L10 (210.82, 137.16) -> (215.9, 137.16)
  line L11 (215.9, 137.16) -> (215.9, 127)
  line L12 (215.9, 106.68) -> (210.82, 106.68)
  line L13 (210.82, 106.68) -> (210.82, 116.84)
  line L14 (210.82, 116.84) -> (215.9, 116.84)
  line L15 (215.9, 116.84) -> (215.9, 106.68)
  line L16 (215.9, 86.36) -> (210.82, 86.36)
  line L17 (210.82, 86.36) -> (210.82, 96.52)
  line L18 (210.82, 96.52) -> (215.9, 96.52)
  line L19 (215.9, 96.52) -> (215.9, 86.36)
  line L20 (215.9, 66.04) -> (210.82, 66.04)
  line L21 (210.82, 66.04) -> (210.82, 76.2)
  line L22 (210.82, 76.2) -> (215.9, 76.2)
  line L23 (215.9, 76.2) -> (215.9, 66.04)
  line L24 (215.9, 45.72) -> (210.82, 45.72)
  line L25 (210.82, 45.72) -> (210.82, 55.88)
  line L26 (210.82, 55.88) -> (215.9, 55.88)
  line L27 (215.9, 55.88) -> (215.9, 45.72)
  line L28 (124.46, 96.52) -> (129.54, 96.52)
  line L29 (124.46, 86.36) -> (124.46, 96.52)
  line L30 (129.54, 96.52) -> (129.54, 86.36)
  line L31 (129.54, 86.36) -> (124.46, 86.36)
  line L32 (124.46, 76.2) -> (129.54, 76.2)
  line L33 (129.54, 66.04) -> (124.46, 66.04)
  line L34 (129.54, 76.2) -> (129.54, 66.04)
  line L35 (124.46, 55.88) -> (129.54, 55.88)
  line L36 (129.54, 45.72) -> (124.46, 45.72)
  line L37 (129.54, 55.88) -> (129.54, 45.72)
  line L38 (124.46, 45.72) -> (124.46, 55.88)
  line L39 (124.46, 66.04) -> (124.46, 76.2)
  line L40 (129.54, 106.68) -> (124.46, 106.68)
  line L41 (124.46, 106.68) -> (124.46, 116.84)
  line L42 (129.54, 116.84) -> (129.54, 106.68)
  line L43 (124.46, 116.84) -> (129.54, 116.84)
  line L44 (129.54, 127) -> (124.46, 127)
  line L45 (124.46, 127) -> (124.46, 137.16)
  line L46 (129.54, 137.16) -> (129.54, 127)
  line L47 (124.46, 137.16) -> (129.54, 137.16)
  line L48 (129.54, 147.32) -> (124.46, 147.32)
  line L49 (124.46, 157.48) -> (129.54, 157.48)
  line L50 (129.54, 157.48) -> (129.54, 147.32)
  line L51 (129.54, 167.64) -> (124.46, 167.64)
  line L52 (124.46, 167.64) -> (124.46, 177.8)
  line L53 (124.46, 177.8) -> (129.54, 177.8)
  line L54 (129.54, 177.8) -> (129.54, 167.64)
  line L55 (124.46, 147.32) -> (124.46, 157.48)
  point P0 (0, 0)
  dimension "d52" = 86.36
  constraints: 112 end point, 15 horizontal, 14 vertical, 1 collinear, 83 other
  measures "d52" distance of L16.start L30.end
extrude "Extrusion6" cut sketch "Sketch5" against normal blind 25.4
sketch "Sketch6" plane through (0, 0, 5.08) normal (0, 0, 1) x (1, 0, 0)
  line L0 (396.0669, 111.578) -> (-133.6623, 111.578)
  line L1 (-133.6623, 111.578) -> (-133.6623, -157.3866)
  line L2 (-133.6623, -157.3866) -> (396.0669, -157.3866)
  line L3 (396.0669, -157.3866) -> (396.0669, 111.578)
  line L4 (215.9, 177.8) -> (215.9, 187.96) projected
  line L5 (215.9, 35.1961) -> (215.9, 187.96)
  point P0 (0, 0)
  point P1 (215.9, 111.578)
  constraints: 10 end point, 2 parallel, 1 horizontal, 1 midpoint, 1 perpendicular, 1 point on line, 1 vertical
extrude "Extrusion7" cut sketch "Sketch6" against normal blind 25.4 keep common part
sketch "Sketch7" plane through (0, 0, 0) normal (0, 0, -1) x (-1, 0, 0)
  line L0 (-83.82, 5.08) -> (-93.98, 5.08)
  line L1 (-93.98, 5.08) -> (-93.98, 0)
  line L2 (-93.98, 0) -> (-83.82, 0)
  line L3 (-83.82, 0) -> (-83.82, 5.08)
  line L4 (-210.82, 111.578) -> (-129.54, 111.578) projected
  line L5 (-210.82, 111.578) -> (-210.82, 106.68) projected
  line L6 (-210.82, 106.68) -> (-215.9, 106.68) projected
  line L7 (-215.9, 106.68) -> (-215.9, 96.52) projected
  line L8 (-215.9, 96.52) -> (-210.82, 96.52) projected
  line L9 (-210.82, 96.52) -> (-210.82, 86.36) projected
  line L10 (-210.82, 86.36) -> (-215.9, 86.36) projected
  line L11 (-215.9, 86.36) -> (-215.9, 76.2) projected
  line L12 (-215.9, 76.2) -> (-210.82, 76.2) projected
  line L13 (-210.82, 76.2) -> (-210.82, 66.04) projected
  line L14 (-210.82, 66.04) -> (-215.9, 66.04) projected
  line L15 (-215.9, 66.04) -> (-215.9, 55.88) projected
  line L16 (-215.9, 55.88) -> (-210.82, 55.88) projected
  line L17 (-210.82, 55.88) -> (-210.82, 45.72) projected
  line L18 (-210.82, 45.72) -> (-215.9, 45.72) projected
  line L19 (-215.9, 45.72) -> (-215.9, 35.56) projected
  line L20 (-215.9, 35.56) -> (-169.545, 9.525) projected
  line L21 (-169.545, 9.525) -> (-147.32, 9.525) projected
  line L22 (-147.32, 9.525) -> (-42.545, -95.25) projected
  line L23 (-42.545, -95.25) -> (-20.32, -95.25) projected
  line L24 (-20.32, -95.25) -> (0, 0) projected
  line L25 (0, 10.16) -> (0, 0) projected
  line L26 (0, 10.16) -> (-5.08, 10.16) projected
  line L27 (-5.08, 10.16) -> (-5.08, 20.32) projected
  line L28 (-5.08, 20.32) -> (0, 20.32) projected
  line L29 (0, 30.48) -> (0, 20.32) projected
  line L30 (0, 30.48) -> (-5.08, 30.48) projected
  line L31 (-5.08, 30.48) -> (-5.08, 40.64) projected
  line L32 (-5.08, 40.64) -> (0, 40.64) projected
  line L33 (0, 50.8) -> (0, 40.64) projected
  line L34 (0, 50.8) -> (-5.08, 50.8) projected
  line L35 (-5.08, 50.8) -> (-5.08, 60.96) projected
  line L36 (-5.08, 60.96) -> (0, 60.96) projected
  line L37 (0, 71.12) -> (0, 60.96) projected
  line L38 (0, 71.12) -> (-5.08, 71.12) projected
  line L39 (-5.08, 71.12) -> (-5.08, 81.28) projected
  line L40 (-5.08, 81.28) -> (0, 81.28) projected
  line L41 (0, 91.44) -> (0, 81.28) projected
  line L42 (0, 91.44) -> (-5.08, 91.44) projected
  line L43 (-5.08, 91.44) -> (-5.08, 101.6) projected
  line L44 (-5.08, 101.6) -> (0, 101.6) projected
  line L45 (0, 111.578) -> (0, 101.6) projected
  line L46 (-124.46, 111.578) -> (0, 111.578) projected
  line L47 (-124.46, 111.578) -> (-124.46, 106.68) projected
  line L48 (-124.46, 106.68) -> (-129.54, 106.68) projected
  line L49 (-129.54, 106.68) -> (-129.54, 111.578) projected
  line L50 (-157.48, 55.245) -> (-157.48, 65.405) projected
  line L51 (-157.48, 65.405) -> (-152.4, 65.405) projected
  line L52 (-152.4, 65.405) -> (-152.4, 55.245) projected
  line L53 (-152.4, 55.245) -> (-157.48, 55.245) projected
  line L54 (-157.48, 34.925) -> (-157.48, 45.085) projected
  line L55 (-157.48, 45.085) -> (-152.4, 45.085) projected
  line L56 (-152.4, 45.085) -> (-152.4, 34.925) projected
  line L57 (-152.4, 34.925) -> (-157.48, 34.925) projected
  line L58 (-157.48, 14.605) -> (-157.48, 24.765) projected
  line L59 (-157.48, 24.765) -> (-152.4, 24.765) projected
  line L60 (-152.4, 24.765) -> (-152.4, 14.605) projected
  line L61 (-152.4, 14.605) -> (-157.48, 14.605) projected
  line L62 (-30.48, -90.17) -> (-30.48, -80.01) projected
  line L63 (-30.48, -80.01) -> (-25.4, -80.01) projected
  line L64 (-25.4, -80.01) -> (-25.4, -90.17) projected
  line L65 (-25.4, -90.17) -> (-30.48, -90.17) projected
  line L66 (-30.48, -59.69) -> (-25.4, -59.69) projected
  line L67 (-25.4, -59.69) -> (-25.4, -69.85) projected
  line L68 (-25.4, -69.85) -> (-30.48, -69.85) projected
  line L69 (-30.48, -69.85) -> (-30.48, -59.69) projected
  line L70 (-30.48, -39.37) -> (-25.4, -39.37) projected
  line L71 (-25.4, -39.37) -> (-25.4, -49.53) projected
  line L72 (-25.4, -49.53) -> (-30.48, -49.53) projected
  line L73 (-30.48, -49.53) -> (-30.48, -39.37) projected
  line L74 (-124.46, 45.72) -> (-129.54, 45.72) projected
  line L75 (-129.54, 45.72) -> (-129.54, 55.88) projected
  line L76 (-129.54, 55.88) -> (-124.46, 55.88) projected
  line L77 (-124.46, 55.88) -> (-124.46, 45.72) projected
  line L78 (-129.54, 86.36) -> (-129.54, 96.52) projected
  line L79 (-129.54, 96.52) -> (-124.46, 96.52) projected
  line L80 (-124.46, 96.52) -> (-124.46, 86.36) projected
  line L81 (-124.46, 86.36) -> (-129.54, 86.36) projected
  line L82 (-129.54, 66.04) -> (-129.54, 76.2) projected
  line L83 (-129.54, 76.2) -> (-124.46, 76.2) projected
  line L84 (-124.46, 76.2) -> (-124.46, 66.04) projected
  line L85 (-124.46, 66.04) -> (-129.54, 66.04) projected
  line L86 (-104.14, 0) -> (-104.14, 5.08)
  line L87 (-114.3, 0) -> (-104.14, 0)
  line L88 (-104.14, 5.08) -> (-114.3, 5.08)
  line L89 (-114.3, 5.08) -> (-114.3, 0)
  line L90 (-124.46, 0) -> (-124.46, 5.08)
  line L91 (-134.62, 0) -> (-124.46, 0)
  line L92 (-124.46, 5.08) -> (-134.62, 5.08)
  line L93 (-134.62, 5.08) -> (-134.62, 0)
  dimension "d59" = 10.16
  dimension "d60" = 5.08
  dimension "d61" = 83.82
  dimension "d62" = 0
  dimension "d65" = 20.32
  constraints: 24 end point, 2 horizontal, 2 parallel, 1 collinear, 1 perpendicular, 15 other
  measures "d59" distance of L1.end L2.end
  measures "d60" distance of L0.end L1.end
  measures "d61" distance from line of L25 L0.start
  measures "d62" distance from line of point (0, 0) L2
  measures "d65" distance of L2.end L86.start
extrude "Extrusion8" cut sketch "Sketch7" against normal blind 25.4 contours L3 L2 L1 L0 | L87 L89 L88 L86 | L91 L93 L92 L90
sketch "Sketch8" plane through (0, 0, 5.08) normal (0, 0, 1) x (1, 0, 0)
  line L0 (140.97, 92.528) -> (140.97, 41.728) construction
  line L1 (133.35, 92.528) -> (133.35, 41.728)
  line L2 (148.59, 41.728) -> (148.59, 92.528)
  arc A0 (148.59, 92.528) -> (133.35, 92.528) centre (140.97, 92.528) ccw
  arc A1 (133.35, 41.728) -> (148.59, 41.728) centre (140.97, 41.728) ccw
  line L3 (104.14, 0) -> (104.14, 5.08) projected
  line L4 (104.14, 5.08) -> (114.3, 5.08) projected
  line L5 (114.3, 5.08) -> (114.3, 0) projected
  line L6 (114.3, 0) -> (104.14, 0) projected
  line L7 (93.98, 5.08) -> (93.98, 0) projected
  line L8 (93.98, 0) -> (83.82, 0) projected
  line L9 (83.82, 0) -> (83.82, 5.08) projected
  line L10 (83.82, 5.08) -> (93.98, 5.08) projected
  line L11 (124.46, 0) -> (124.46, 5.08) projected
  line L12 (124.46, 5.08) -> (134.62, 5.08) projected
  line L13 (134.62, 5.08) -> (134.62, 0) projected
  line L14 (134.62, 0) -> (124.46, 0) projected
  line L15 (157.48, 65.405) -> (157.48, 55.245) projected
  line L16 (157.48, 55.245) -> (152.4, 55.245) projected
  line L17 (152.4, 55.245) -> (152.4, 65.405) projected
  line L18 (152.4, 65.405) -> (157.48, 65.405) projected
  line L19 (157.48, 45.085) -> (157.48, 34.925) projected
  line L20 (157.48, 34.925) -> (152.4, 34.925) projected
  line L21 (152.4, 34.925) -> (152.4, 45.085) projected
  line L22 (152.4, 45.085) -> (157.48, 45.085) projected
  line L23 (157.48, 24.765) -> (157.48, 14.605) projected
  line L24 (157.48, 14.605) -> (152.4, 14.605) projected
  line L25 (152.4, 14.605) -> (152.4, 24.765) projected
  line L26 (152.4, 24.765) -> (157.48, 24.765) projected
  line L27 (30.48, -80.01) -> (30.48, -90.17) projected
  line L28 (30.48, -90.17) -> (25.4, -90.17) projected
  line L29 (25.4, -90.17) -> (25.4, -80.01) projected
  line L30 (25.4, -80.01) -> (30.48, -80.01) projected
  line L31 (25.4, -59.69) -> (30.48, -59.69) projected
  line L32 (30.48, -59.69) -> (30.48, -69.85) projected
  line L33 (30.48, -69.85) -> (25.4, -69.85) projected
  line L34 (25.4, -69.85) -> (25.4, -59.69) projected
  line L35 (25.4, -39.37) -> (30.48, -39.37) projected
  line L36 (30.48, -39.37) -> (30.48, -49.53) projected
  line L37 (30.48, -49.53) -> (25.4, -49.53) projected
  line L38 (25.4, -49.53) -> (25.4, -39.37) projected
  line L39 (129.54, 45.72) -> (124.46, 45.72) projected
  line L40 (124.46, 45.72) -> (124.46, 55.88) projected
  line L41 (124.46, 55.88) -> (129.54, 55.88) projected
  line L42 (129.54, 55.88) -> (129.54, 45.72) projected
  line L43 (129.54, 96.52) -> (129.54, 86.36) projected
  line L44 (129.54, 86.36) -> (124.46, 86.36) projected
  line L45 (124.46, 86.36) -> (124.46, 96.52) projected
  line L46 (124.46, 96.52) -> (129.54, 96.52) projected
  line L47 (129.54, 76.2) -> (129.54, 66.04) projected
  line L48 (129.54, 66.04) -> (124.46, 66.04) projected
  line L49 (124.46, 66.04) -> (124.46, 76.2) projected
  line L50 (124.46, 76.2) -> (129.54, 76.2) projected
  line L51 (129.54, 111.578) -> (210.82, 111.578) projected
  line L52 (129.54, 111.578) -> (129.54, 106.68) projected
  line L53 (129.54, 106.68) -> (124.46, 106.68) projected
  line L54 (124.46, 106.68) -> (124.46, 111.578) projected
  line L55 (0, 111.578) -> (124.46, 111.578) projected
  line L56 (0, 111.578) -> (0, 101.6) projected
  line L57 (0, 101.6) -> (5.08, 101.6) projected
  line L58 (5.08, 101.6) -> (5.08, 91.44) projected
  line L59 (5.08, 91.44) -> (0, 91.44) projected
  line L60 (0, 91.44) -> (0, 81.28) projected
  line L61 (0, 81.28) -> (5.08, 81.28) projected
  line L62 (5.08, 81.28) -> (5.08, 71.12) projected
  line L63 (5.08, 71.12) -> (0, 71.12) projected
  line L64 (0, 71.12) -> (0, 60.96) projected
  line L65 (0, 60.96) -> (5.08, 60.96) projected
  line L66 (5.08, 60.96) -> (5.08, 50.8) projected
  line L67 (5.08, 50.8) -> (0, 50.8) projected
  line L68 (0, 50.8) -> (0, 40.64) projected
  line L69 (0, 40.64) -> (5.08, 40.64) projected
  line L70 (5.08, 40.64) -> (5.08, 30.48) projected
  line L71 (5.08, 30.48) -> (0, 30.48) projected
  line L72 (0, 30.48) -> (0, 20.32) projected
  line L73 (0, 20.32) -> (5.08, 20.32) projected
  line L74 (5.08, 20.32) -> (5.08, 10.16) projected
  line L75 (5.08, 10.16) -> (0, 10.16) projected
  line L76 (0, 10.16) -> (0, 0) projected
  line L77 (0, 0) -> (20.32, -95.25) projected
  line L78 (20.32, -95.25) -> (42.545, -95.25) projected
  line L79 (42.545, -95.25) -> (147.32, 9.525) projected
  line L80 (147.32, 9.525) -> (169.545, 9.525) projected
  line L81 (169.545, 9.525) -> (215.9, 35.56) projected
  line L82 (215.9, 35.56) -> (215.9, 45.72) projected
  line L83 (215.9, 45.72) -> (210.82, 45.72) projected
  line L84 (210.82, 45.72) -> (210.82, 55.88) projected
  line L85 (210.82, 55.88) -> (215.9, 55.88) projected
  line L86 (215.9, 55.88) -> (215.9, 66.04) projected
  line L87 (215.9, 66.04) -> (210.82, 66.04) projected
  line L88 (210.82, 66.04) -> (210.82, 76.2) projected
  line L89 (210.82, 76.2) -> (215.9, 76.2) projected
  line L90 (215.9, 76.2) -> (215.9, 86.36) projected
  line L91 (215.9, 86.36) -> (210.82, 86.36) projected
  line L92 (210.82, 86.36) -> (210.82, 96.52) projected
  line L93 (210.82, 96.52) -> (215.9, 96.52) projected
  line L94 (215.9, 96.52) -> (215.9, 106.68) projected
  line L95 (215.9, 106.68) -> (210.82, 106.68) projected
  line L96 (210.82, 106.68) -> (210.82, 111.578) projected
  point P0 (140.97, 67.128)
  dimension "d72" = 7.62
  dimension "d73" = 22.86
  dimension "d74" = 11.43
  dimension "d75" = 50.8
  dimension "d76" = 19.05
  constraints: 8 end point, 4 point on circle, 4 tangent, 2 centre point, 1 midpoint, 1 parallel, 1 vertical
  measures "d72" radius of A1
  measures "d73" distance between parallel lines of L42 L17
  measures "d74" distance between parallel lines of L0 L17
  measures "d75" distance of L0.start L0.end
  measures "d76" distance from line of L51 L0.start
extrude "Extrusion9" cut sketch "Sketch8" against normal blind 25.4 contours A0 L2 A1 L1